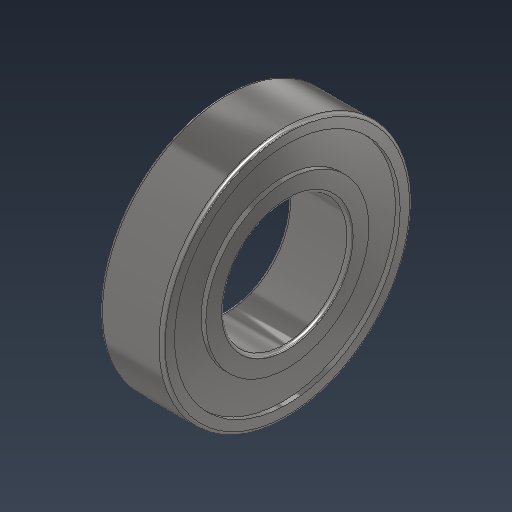
# Autodesk Inventor part: B6901ZZ
Saved by Autodesk Inventor 2021 (Build 250183000, 183)
## iProperties
Category: PARTsolutions
Company: MISUMI
Part Number: B6901ZZ
Material: 鋼、炭素鋼
Catalog Web Link: www.cadenas.de
Description: ミスミ
Vendor: MISUMI
Document SubType Name: Modeling
Designer: partserver
Manufacturer: MISUMI
Mass: 14.7079 g
Surface Area: 14.3322 cm^2
Volume: 1.87361 cm^3
Density: 7.85 g/cm^3
Appearance: 半つや出し
PSOL_IDENT_0: {$CADENAS_DATA\23d-libs\misumi\metric\12_bearing_holders\sb6010zz.prj},171 {VTYP=3D},{NB=B6901ZZ},{L
PSOL_IDENT_1: INA=B6901ZZ},{NN=B6_ _ _ZZ, SB6_ _ _ZZ},{DATE=30.10.2020 16:03:36},{GEOMDATE=22.10.2019 06:26:04},{V
PSOL_IDENT_2: ERSION=},{LINEID=80},{WBVAR=TS},{WBNUMERIC=}  {NB=B6901ZZ},{LINA=B6901ZZ},{KT=DUMMY},{PN=B6901ZZ},{T
PSOL_IDENT_3: S=},{TS1= '', 'Steel', 'S', 'Stainless Steel'},{MAT=52100 Bearing Steel},{BN=6901ZZ},{DD=12},{D=24},
PSOL_IDENT_4: {B=6},{RR=0.3},{CR=2.89},{COR=1.46},{CRS=2.89},{CRSS=2.45},{CORS=1.46},{CORSS=1.18},{DD1=22.80},{R1=
PSOL_IDENT_5: 0.20},{R2=0.3},{DSMIN=14.0},{DSMAX=15.00},{DS1=15.00},{DDHH=22.0},{R=0.3},{MASS=11},{MASS11=11},{AA=
PSOL_IDENT_6: 5.1000},{BB=1.2000},{CC=1.8000},{TYS=w/o Retaining Ring}
NB: B6901ZZ
NN: B6_ _ _ZZ, SB6_ _ _ZZ
NT: Deep Groove Ball Bearings - Double Shield Type
NBSYN: $PN.
LINA: B6901ZZ
CATALOG: Misumi
PN: B6901ZZ
TS: Steel
MAT: 52100 Bearing Steel
BN: 6901ZZ
DD: 12
D: 24
B: 6
RR: 0.3
CR: 2.89
COR: 1.46
DSMIN: 14
DSMAX: 15
DDHH: 22
R: 0.3
MASS: 11
SUPPLIER: MISUMI
ARTICLENO: B6901ZZ
BOMINFO: B6901ZZ
CREATOR: CADENAS GmbH
Title: B6901ZZ
Author: Cadenas PARTsolutions
Comments: Deep Groove Ball Bearings - Double Shield Type
Autodesk Inventor part; units mm, degrees
sketch "Sketch_1" plane through (0, 0, 0) normal (0, 0, 1) x (1, 0, 0)
  line L0 (6, 0) -> (0, 0)
  arc A0 (0, 6.3) -> (0.3, 6) centre (0.3, 6.3) ccw
  line L1 (0.3, 6) -> (5.7, 6)
  arc A1 (5.7, 6) -> (6, 6.3) centre (5.7, 6.3) ccw
  line L2 (6, 6.3) -> (6, 7.8)
  line L3 (6, 7.8) -> (5.55, 7.8)
  line L4 (5.55, 7.8) -> (5.55, 10.8)
  line L5 (5.55, 10.8) -> (6, 10.8)
  line L6 (6, 10.8) -> (6, 11.7)
  arc A2 (6, 11.7) -> (5.7, 12) centre (5.7, 11.7) ccw
  line L7 (5.7, 12) -> (0.3, 12)
  arc A3 (0.3, 12) -> (0, 11.7) centre (0.3, 11.7) ccw
  line L8 (0, 11.7) -> (0, 10.8)
  line L9 (0, 10.8) -> (0.45, 10.8)
  line L10 (0.45, 10.8) -> (0.45, 7.8)
  line L11 (0.45, 7.8) -> (0, 7.8)
  line L12 (0, 7.8) -> (0, 6.3)
  constraints: 26 end point, 8 point on circle, 4 centre point
revolve "Revolution1" add sketch "Sketch_1" angle 360 about axis through (6, 0, 0) along (1, 0, 0)
ref_plane "center_point_XY" through (3, 0, 0) normal (1, 0, 0) x (0, 0, -1)
ref_plane "center_point_YZ" through (3, 0, 0) normal (0, 0, -1) x (0, 1, 0)
ref_plane "center_point_ZX" through (3, 0, 0) normal (0, 1, 0) x (1, 0, 0)
ref_plane "to_housing_XY" through (0, 0, 0) normal (1, 0, 0) x (0, 0, -1)
ref_plane "to_housing_YZ" through (0, 0, 0) normal (0, 0, -1) x (0, 1, 0)
ref_plane "to_housing_ZX" through (0, 0, 0) normal (0, 1, 0) x (1, 0, 0)
ref_plane "to_ring_XY" through (5.1, 0, 0) normal (1, 0, 0) x (0, 0, -1)
ref_plane "to_ring_YZ" through (5.1, 0, 0) normal (0, 0, -1) x (0, 1, 0)
ref_plane "to_ring_ZX" through (5.1, 0, 0) normal (0, 1, 0) x (1, 0, 0)
body "Solid1"
